Autodesk Fusion 360 part; units mm, degrees
(part 9 of 10)
equation "d1708 = PegSize + 2 * FitClearance"
equation "d1709 = PegSize + 2 * FitClearance"
equation "d1710 = PegHeight + 0.3 mm"
equation "d1712 = FootHeight"
equation "d1714 = ( BaseX + LeftRun + FaucetGap + RightRun - RightSideDepth ) + ( ( RightSideDepth ) - ( ( ( ( RightSideDepth ) - FrontFootInset ) - PegSize / 2 - FitClearance ) + ( PegSize + 2 * FitClearance ) ) )"
equation "d1715 = ( BaseY + Depth + ModuleGap ) + ( ( 11 mm ) - PegSize / 2 - FitClearance )"
equation "d1716 = PegSize + 2 * FitClearance"
equation "d1717 = PegSize + 2 * FitClearance"
equation "d1718 = PegHeight + 0.3 mm"
equation "d1720 = FootHeight"
equation "d1722 = ( BaseX + LeftRun + FaucetGap + RightRun - RightSideDepth ) + ( ( RightSideDepth ) - ( ( ( 11 mm ) - PegSize / 2 - FitClearance ) + ( PegSize + 2 * FitClearance ) ) )"
equation "d1723 = ( BaseY + Depth + ModuleGap ) + ( ( ( RightReach ) - 11 mm ) - PegSize / 2 - FitClearance )"
equation "d1724 = PegSize + 2 * FitClearance"
equation "d1725 = PegSize + 2 * FitClearance"
equation "d1726 = PegHeight + 0.3 mm"
equation "d1728 = FootHeight"
equation "d1730 = ( BaseX + LeftRun + FaucetGap + RightRun - RightSideDepth ) + ( ( RightSideDepth ) - ( ( ( ( RightSideDepth ) - FrontFootInset ) - PegSize / 2 - FitClearance ) + ( PegSize + 2 * FitClearance ) ) )"
equation "d1731 = ( BaseY + Depth + ModuleGap ) + ( ( ( RightReach ) - 11 mm ) - PegSize / 2 - FitClearance )"
equation "d1732 = PegSize + 2 * FitClearance"
equation "d1733 = PegSize + 2 * FitClearance"
equation "d1734 = PegHeight + 0.3 mm"
equation "d1736 = ( FootHeight ) + PanHeight - DeckThick"
equation "d1738 = ( BaseX + LeftRun + FaucetGap + RightRun - RightSideDepth ) + ( ( RightSideDepth ) - ( ( Wall + DeckClearance ) + ( ( RightSideDepth ) - 2 * ( Wall + DeckClearance ) ) ) )"
equation "d1739 = ( BaseY + Depth + ModuleGap ) + ( Wall + DeckClearance )"
equation "d1740 = ( RightSideDepth ) - 2 * ( Wall + DeckClearance )"
equation "d1741 = ( RightReach ) - 2 * ( Wall + DeckClearance )"
equation "d1742 = DeckThick"
equation "d1744 = ( FootHeight ) + PanHeight - DeckThick"
equation "d1746 = ( BaseX + LeftRun + FaucetGap + RightRun - RightSideDepth ) + ( ( RightSideDepth ) - ( ( Wall + DeckClearance + RimBorder ) + ( ( RightSideDepth ) - 2 * ( Wall + DeckClearance + RimBorder ) ) ) )"
equation "d1747 = ( BaseY + Depth + ModuleGap ) + ( ( ( ( RightReach ) - ( 14 * SlotPitch + SlotWidth ) ) / 2 ) + ( 0 * SlotPitch ) )"
equation "d1748 = ( RightSideDepth ) - 2 * ( Wall + DeckClearance + RimBorder )"
equation "d1749 = SlotWidth"
equation "d1750 = DeckThick"
equation "d1752 = ( FootHeight ) + PanHeight - DeckThick"
equation "d1754 = ( BaseX + LeftRun + FaucetGap + RightRun - RightSideDepth ) + ( ( RightSideDepth ) - ( ( Wall + DeckClearance + RimBorder ) + ( ( RightSideDepth ) - 2 * ( Wall + DeckClearance + RimBorder ) ) ) )"
equation "d1755 = ( BaseY + Depth + ModuleGap ) + ( ( ( ( RightReach ) - ( 14 * SlotPitch + SlotWidth ) ) / 2 ) + ( 1 * SlotPitch ) )"
equation "d1756 = ( RightSideDepth ) - 2 * ( Wall + DeckClearance + RimBorder )"
equation "d1757 = SlotWidth"
equation "d1758 = DeckThick"
equation "d1760 = ( FootHeight ) + PanHeight - DeckThick"
equation "d1762 = ( BaseX + LeftRun + FaucetGap + RightRun - RightSideDepth ) + ( ( RightSideDepth ) - ( ( Wall + DeckClearance + RimBorder ) + ( ( RightSideDepth ) - 2 * ( Wall + DeckClearance + RimBorder ) ) ) )"
equation "d1763 = ( BaseY + Depth + ModuleGap ) + ( ( ( ( RightReach ) - ( 14 * SlotPitch + SlotWidth ) ) / 2 ) + ( 2 * SlotPitch ) )"
equation "d1764 = ( RightSideDepth ) - 2 * ( Wall + DeckClearance + RimBorder )"
equation "d1765 = SlotWidth"
equation "d1766 = DeckThick"
equation "d1768 = ( FootHeight ) + PanHeight - DeckThick"
equation "d1770 = ( BaseX + LeftRun + FaucetGap + RightRun - RightSideDepth ) + ( ( RightSideDepth ) - ( ( Wall + DeckClearance + RimBorder ) + ( ( RightSideDepth ) - 2 * ( Wall + DeckClearance + RimBorder ) ) ) )"
equation "d1771 = ( BaseY + Depth + ModuleGap ) + ( ( ( ( RightReach ) - ( 14 * SlotPitch + SlotWidth ) ) / 2 ) + ( 3 * SlotPitch ) )"
equation "d1772 = ( RightSideDepth ) - 2 * ( Wall + DeckClearance + RimBorder )"
equation "d1773 = SlotWidth"
equation "d1774 = DeckThick"
equation "d1776 = ( FootHeight ) + PanHeight - DeckThick"
equation "d1778 = ( BaseX + LeftRun + FaucetGap + RightRun - RightSideDepth ) + ( ( RightSideDepth ) - ( ( Wall + DeckClearance + RimBorder ) + ( ( RightSideDepth ) - 2 * ( Wall + DeckClearance + RimBorder ) ) ) )"
equation "d1779 = ( BaseY + Depth + ModuleGap ) + ( ( ( ( RightReach ) - ( 14 * SlotPitch + SlotWidth ) ) / 2 ) + ( 4 * SlotPitch ) )"
equation "d1780 = ( RightSideDepth ) - 2 * ( Wall + DeckClearance + RimBorder )"
equation "d1781 = SlotWidth"
equation "d1782 = DeckThick"
equation "d1784 = ( FootHeight ) + PanHeight - DeckThick"
equation "d1786 = ( BaseX + LeftRun + FaucetGap + RightRun - RightSideDepth ) + ( ( RightSideDepth ) - ( ( Wall + DeckClearance + RimBorder ) + ( ( RightSideDepth ) - 2 * ( Wall + DeckClearance + RimBorder ) ) ) )"
equation "d1787 = ( BaseY + Depth + ModuleGap ) + ( ( ( ( RightReach ) - ( 14 * SlotPitch + SlotWidth ) ) / 2 ) + ( 5 * SlotPitch ) )"
equation "d1788 = ( RightSideDepth ) - 2 * ( Wall + DeckClearance + RimBorder )"
equation "d1789 = SlotWidth"
equation "d1790 = DeckThick"
equation "d1792 = ( FootHeight ) + PanHeight - DeckThick"
equation "d1794 = ( BaseX + LeftRun + FaucetGap + RightRun - RightSideDepth ) + ( ( RightSideDepth ) - ( ( Wall + DeckClearance + RimBorder ) + ( ( RightSideDepth ) - 2 * ( Wall + DeckClearance + RimBorder ) ) ) )"
equation "d1795 = ( BaseY + Depth + ModuleGap ) + ( ( ( ( RightReach ) - ( 14 * SlotPitch + SlotWidth ) ) / 2 ) + ( 6 * SlotPitch ) )"
equation "d1796 = ( RightSideDepth ) - 2 * ( Wall + DeckClearance + RimBorder )"
equation "d1797 = SlotWidth"
equation "d1798 = DeckThick"
equation "d1800 = ( FootHeight ) + PanHeight - DeckThick"
equation "d1802 = ( BaseX + LeftRun + FaucetGap + RightRun - RightSideDepth ) + ( ( RightSideDepth ) - ( ( Wall + DeckClearance + RimBorder ) + ( ( RightSideDepth ) - 2 * ( Wall + DeckClearance + RimBorder ) ) ) )"
equation "d1803 = ( BaseY + Depth + ModuleGap ) + ( ( ( ( RightReach ) - ( 14 * SlotPitch + SlotWidth ) ) / 2 ) + ( 7 * SlotPitch ) )"
equation "d1804 = ( RightSideDepth ) - 2 * ( Wall + DeckClearance + RimBorder )"
equation "d1805 = SlotWidth"
equation "d1806 = DeckThick"
equation "d1808 = ( FootHeight ) + PanHeight - DeckThick"
equation "d1810 = ( BaseX + LeftRun + FaucetGap + RightRun - RightSideDepth ) + ( ( RightSideDepth ) - ( ( Wall + DeckClearance + RimBorder ) + ( ( RightSideDepth ) - 2 * ( Wall + DeckClearance + RimBorder ) ) ) )"
equation "d1811 = ( BaseY + Depth + ModuleGap ) + ( ( ( ( RightReach ) - ( 14 * SlotPitch + SlotWidth ) ) / 2 ) + ( 8 * SlotPitch ) )"
equation "d1812 = ( RightSideDepth ) - 2 * ( Wall + DeckClearance + RimBorder )"
equation "d1813 = SlotWidth"
equation "d1814 = DeckThick"
equation "d1816 = ( FootHeight ) + PanHeight - DeckThick"
equation "d1818 = ( BaseX + LeftRun + FaucetGap + RightRun - RightSideDepth ) + ( ( RightSideDepth ) - ( ( Wall + DeckClearance + RimBorder ) + ( ( RightSideDepth ) - 2 * ( Wall + DeckClearance + RimBorder ) ) ) )"
equation "d1819 = ( BaseY + Depth + ModuleGap ) + ( ( ( ( RightReach ) - ( 14 * SlotPitch + SlotWidth ) ) / 2 ) + ( 9 * SlotPitch ) )"
equation "d1820 = ( RightSideDepth ) - 2 * ( Wall + DeckClearance + RimBorder )"
equation "d1821 = SlotWidth"
equation "d1822 = DeckThick"
equation "d1824 = ( FootHeight ) + PanHeight - DeckThick"
equation "d1826 = ( BaseX + LeftRun + FaucetGap + RightRun - RightSideDepth ) + ( ( RightSideDepth ) - ( ( Wall + DeckClearance + RimBorder ) + ( ( RightSideDepth ) - 2 * ( Wall + DeckClearance + RimBorder ) ) ) )"
equation "d1827 = ( BaseY + Depth + ModuleGap ) + ( ( ( ( RightReach ) - ( 14 * SlotPitch + SlotWidth ) ) / 2 ) + ( 10 * SlotPitch ) )"
equation "d1828 = ( RightSideDepth ) - 2 * ( Wall + DeckClearance + RimBorder )"
equation "d1829 = SlotWidth"
equation "d1830 = DeckThick"
equation "d1832 = ( FootHeight ) + PanHeight - DeckThick"
equation "d1834 = ( BaseX + LeftRun + FaucetGap + RightRun - RightSideDepth ) + ( ( RightSideDepth ) - ( ( Wall + DeckClearance + RimBorder ) + ( ( RightSideDepth ) - 2 * ( Wall + DeckClearance + RimBorder ) ) ) )"
equation "d1835 = ( BaseY + Depth + ModuleGap ) + ( ( ( ( RightReach ) - ( 14 * SlotPitch + SlotWidth ) ) / 2 ) + ( 11 * SlotPitch ) )"
equation "d1836 = ( RightSideDepth ) - 2 * ( Wall + DeckClearance + RimBorder )"
equation "d1837 = SlotWidth"
equation "d1838 = DeckThick"
equation "d1840 = ( FootHeight ) + PanHeight - DeckThick"
equation "d1842 = ( BaseX + LeftRun + FaucetGap + RightRun - RightSideDepth ) + ( ( RightSideDepth ) - ( ( Wall + DeckClearance + RimBorder ) + ( ( RightSideDepth ) - 2 * ( Wall + DeckClearance + RimBorder ) ) ) )"
equation "d1843 = ( BaseY + Depth + ModuleGap ) + ( ( ( ( RightReach ) - ( 14 * SlotPitch + SlotWidth ) ) / 2 ) + ( 12 * SlotPitch ) )"
equation "d1844 = ( RightSideDepth ) - 2 * ( Wall + DeckClearance + RimBorder )"
equation "d1845 = SlotWidth"
equation "d1846 = DeckThick"
equation "d1848 = ( FootHeight ) + PanHeight - DeckThick"
equation "d1850 = ( BaseX + LeftRun + FaucetGap + RightRun - RightSideDepth ) + ( ( RightSideDepth ) - ( ( Wall + DeckClearance + RimBorder ) + ( ( RightSideDepth ) - 2 * ( Wall + DeckClearance + RimBorder ) ) ) )"
equation "d1851 = ( BaseY + Depth + ModuleGap ) + ( ( ( ( RightReach ) - ( 14 * SlotPitch + SlotWidth ) ) / 2 ) + ( 13 * SlotPitch ) )"
equation "d1852 = ( RightSideDepth ) - 2 * ( Wall + DeckClearance + RimBorder )"
equation "d1853 = SlotWidth"
equation "d1854 = DeckThick"
equation "d1856 = ( FootHeight ) + PanHeight - DeckThick"
equation "d1858 = ( BaseX + LeftRun + FaucetGap + RightRun - RightSideDepth ) + ( ( RightSideDepth ) - ( ( Wall + DeckClearance + RimBorder ) + ( ( RightSideDepth ) - 2 * ( Wall + DeckClearance + RimBorder ) ) ) )"
equation "d1859 = ( BaseY + Depth + ModuleGap ) + ( ( ( ( RightReach ) - ( 14 * SlotPitch + SlotWidth ) ) / 2 ) + ( 14 * SlotPitch ) )"
equation "d1860 = ( RightSideDepth ) - 2 * ( Wall + DeckClearance + RimBorder )"
equation "d1861 = SlotWidth"
equation "d1862 = DeckThick"
equation "d1864 = ( FootHeight ) + PanHeight - DeckThick"
equation "d1866 = ( BaseX + LeftRun + FaucetGap + RightRun - RightSideDepth ) + ( ( RightSideDepth ) - ( ( ( RightSideDepth ) - Wall - DeckClearance - 4 mm ) + ( 5 mm ) ) )"
equation "d1867 = ( BaseY + Depth + ModuleGap ) + ( ( RightReach ) / 2 - 8 mm )"
equation "d1870 = DeckThick"
equation "d1874 = ( BaseX + LeftRun + FaucetGap + RightRun - RightSideDepth ) + ( ( RightSideDepth ) - ( ( ( 11 mm ) - FootSize / 2 ) + ( FootSize ) ) )"
equation "d1875 = ( BaseY + Depth + ModuleGap ) + ( ( 11 mm ) - FootSize / 2 )"
equation "d1876 = FootSize"
equation "d1877 = FootSize"
equation "d1878 = FootHeight"
equation "d1880 = FootHeight"
equation "d1882 = ( BaseX + LeftRun + FaucetGap + RightRun - RightSideDepth ) + ( ( RightSideDepth ) - ( ( ( 11 mm ) - PegSize / 2 ) + ( PegSize ) ) )"
equation "d1883 = ( BaseY + Depth + ModuleGap ) + ( ( 11 mm ) - PegSize / 2 )"
equation "d1884 = PegSize"
equation "d1885 = PegSize"
equation "d1886 = PegHeight"
equation "d1890 = ( BaseX + LeftRun + FaucetGap + RightRun - RightSideDepth ) + ( ( RightSideDepth ) - ( ( ( ( RightSideDepth ) - FrontFootInset ) - FootSize / 2 ) + ( FootSize ) ) )"
equation "d1891 = ( BaseY + Depth + ModuleGap ) + ( ( 11 mm ) - FootSize / 2 )"
equation "d1892 = FootSize"
equation "d1893 = FootSize"
equation "d1894 = FootHeight"
equation "d1896 = FootHeight"
equation "d1898 = ( BaseX + LeftRun + FaucetGap + RightRun - RightSideDepth ) + ( ( RightSideDepth ) - ( ( ( ( RightSideDepth ) - FrontFootInset ) - PegSize / 2 ) + ( PegSize ) ) )"
equation "d1899 = ( BaseY + Depth + ModuleGap ) + ( ( 11 mm ) - PegSize / 2 )"
equation "d1900 = PegSize"
equation "d1901 = PegSize"
equation "d1902 = PegHeight"
equation "d1906 = ( BaseX + LeftRun + FaucetGap + RightRun - RightSideDepth ) + ( ( RightSideDepth ) - ( ( ( 11 mm ) - FootSize / 2 ) + ( FootSize ) ) )"
equation "d1907 = ( BaseY + Depth + ModuleGap ) + ( ( ( RightReach ) - 11 mm ) - FootSize / 2 )"
equation "d1908 = FootSize"
equation "d1909 = FootSize"
equation "d1910 = FootHeight"
equation "d1912 = FootHeight"
equation "d1914 = ( BaseX + LeftRun + FaucetGap + RightRun - RightSideDepth ) + ( ( RightSideDepth ) - ( ( ( 11 mm ) - PegSize / 2 ) + ( PegSize ) ) )"
equation "d1915 = ( BaseY + Depth + ModuleGap ) + ( ( ( RightReach ) - 11 mm ) - PegSize / 2 )"
equation "d1916 = PegSize"
equation "d1917 = PegSize"
equation "d1918 = PegHeight"
equation "d1922 = ( BaseX + LeftRun + FaucetGap + RightRun - RightSideDepth ) + ( ( RightSideDepth ) - ( ( ( ( RightSideDepth ) - FrontFootInset ) - FootSize / 2 ) + ( FootSize ) ) )"
equation "d1923 = ( BaseY + Depth + ModuleGap ) + ( ( ( RightReach ) - 11 mm ) - FootSize / 2 )"
equation "d1924 = FootSize"
equation "d1925 = FootSize"
equation "d1926 = FootHeight"
equation "d1928 = FootHeight"
equation "d1930 = ( BaseX + LeftRun + FaucetGap + RightRun - RightSideDepth ) + ( ( RightSideDepth ) - ( ( ( ( RightSideDepth ) - FrontFootInset ) - PegSize / 2 ) + ( PegSize ) ) )"
equation "d1931 = ( BaseY + Depth + ModuleGap ) + ( ( ( RightReach ) - 11 mm ) - PegSize / 2 )"
equation "d1932 = PegSize"
equation "d1933 = PegSize"
equation "d1934 = PegHeight"
equation "d1936 = UpperDeckHeight - PanHeight"
equation "d1938 = ( BaseX ) + ( 0 mm )"
equation "d1939 = ( BaseY ) + ( 0 mm )"
equation "d1940 = TowerWidth"
equation "d1941 = Depth"
equation "d1942 = PanHeight"
equation "d1946 = ( BaseX ) + ( Wall )"
equation "d1948 = -( -( ( UpperDeckHeight - PanHeight ) + FloorMin + DrainExtension * tan(DrainSlope) + ( ( Depth ) - ( Wall ) ) * tan(DrainSlope) ) )"
equation "d1949 = ( ( BaseY ) + ( Wall ) )"
equation "d1950 = -( -( ( UpperDeckHeight - PanHeight ) + FloorMin + DrainExtension * tan(DrainSlope) + ( ( Depth ) - ( ( Depth ) - Wall ) ) * tan(DrainSlope) ) )"
equation "d1951 = ( ( BaseY ) + ( ( Depth ) - Wall ) )"
equation "d1952 = -( -( ( UpperDeckHeight - PanHeight ) + PanHeight + 1 mm ) )"
equation "d1953 = ( TowerWidth ) - 2 * Wall"
equation "d1955 = ( BaseX ) + ( ( TowerWidth - 35 mm ) - DrainWidth / 2 - Wall )"
equation "d1957 = -( -( UpperDeckHeight - PanHeight ) )"
equation "d1958 = ( ( BaseY ) + ( ( Depth ) - Wall ) )"
equation "d1959 = ( ( BaseY ) + ( ( Depth ) + DrainExtension ) )"
equation "d1960 = -( -( ( UpperDeckHeight - PanHeight ) + FloorMin + DrainExtension * tan(DrainSlope) + ( ( Depth ) - ( ( Depth ) + DrainExtension ) ) * tan(DrainSlope) ) )"
equation "d1961 = -( -( ( UpperDeckHeight - PanHeight ) + FloorMin + DrainExtension * tan(DrainSlope) + ( ( Depth ) - ( ( Depth ) - Wall ) ) * tan(DrainSlope) ) )"
equation "d1962 = DrainWidth + 2 * Wall"
equation "d1964 = ( BaseX ) + ( ( TowerWidth - 35 mm ) - DrainWidth / 2 - Wall )"
equation "d1966 = -( -( UpperDeckHeight - PanHeight ) )"
equation "d1967 = ( ( BaseY ) + ( ( Depth ) - Wall ) )"
equation "d1968 = ( ( BaseY ) + ( ( Depth ) + DrainExtension ) )"
equation "d1969 = -( -( ( ( UpperDeckHeight - PanHeight ) + FloorMin + DrainExtension * tan(DrainSlope) + ( ( Depth ) - ( ( Depth ) + DrainExtension ) ) * tan(DrainSlope) ) + ( 6 mm ) ) )"
equation "d1970 = -( -( ( ( UpperDeckHeight - PanHeight ) + FloorMin + DrainExtension * tan(DrainSlope) + ( ( Depth ) - ( ( Depth ) - Wall ) ) * tan(DrainSlope) ) + ( 6 mm ) ) )"
equation "d1971 = Wall"
equation "d1973 = ( BaseX ) + ( ( TowerWidth - 35 mm ) + DrainWidth / 2 )"
equation "d1975 = -( -( UpperDeckHeight - PanHeight ) )"
equation "d1976 = ( ( BaseY ) + ( ( Depth ) - Wall ) )"
equation "d1977 = ( ( BaseY ) + ( ( Depth ) + DrainExtension ) )"
equation "d1978 = -( -( ( ( UpperDeckHeight - PanHeight ) + FloorMin + DrainExtension * tan(DrainSlope) + ( ( Depth ) - ( ( Depth ) + DrainExtension ) ) * tan(DrainSlope) ) + ( 6 mm ) ) )"
equation "d1979 = -( -( ( ( UpperDeckHeight - PanHeight ) + FloorMin + DrainExtension * tan(DrainSlope) + ( ( Depth ) - ( ( Depth ) - Wall ) ) * tan(DrainSlope) ) + ( 6 mm ) ) )"
equation "d1980 = Wall"
equation "d1982 = ( BaseX ) + ( ( TowerWidth - 35 mm ) - DrainWidth / 2 )"
equation "d1984 = -( -( ( UpperDeckHeight - PanHeight ) + FloorMin + DrainExtension * tan(DrainSlope) + ( ( Depth ) - ( ( Depth ) - Wall ) ) * tan(DrainSlope) ) )"
equation "d1985 = ( ( BaseY ) + ( ( Depth ) - Wall ) )"
equation "d1986 = -( -( ( UpperDeckHeight - PanHeight ) + FloorMin + DrainExtension * tan(DrainSlope) + ( ( Depth ) - ( ( Depth ) + DrainExtension ) ) * tan(DrainSlope) ) )"
equation "d1987 = ( ( BaseY ) + ( ( Depth ) + DrainExtension ) )"
equation "d1988 = -( -( ( UpperDeckHeight - PanHeight ) + PanHeight + 1 mm ) )"
equation "d1989 = DrainWidth"
equation "d1991 = UpperDeckHeight - PanHeight"
equation "d1993 = ( BaseX ) + ( Wall )"
equation "d1994 = ( BaseY ) + ( Wall )"
equation "d1997 = PanHeight - DeckThick"
equation "d1999 = UpperDeckHeight - PanHeight"
equation "d2001 = ( BaseX ) + ( Wall )"
equation "d2002 = ( BaseY ) + ( ( Depth ) - Wall - 12 mm )"
equation "d2005 = PanHeight - DeckThick"
equation "d2007 = UpperDeckHeight - PanHeight"
equation "d2009 = ( BaseX ) + ( ( TowerWidth ) - Wall - 12 mm )"
equation "d2010 = ( BaseY ) + ( Wall )"
equation "d2013 = PanHeight - DeckThick"
equation "d2015 = UpperDeckHeight - PanHeight"
equation "d2017 = ( BaseX ) + ( ( TowerWidth ) - Wall - 12 mm )"
equation "d2018 = ( BaseY ) + ( ( Depth ) - Wall - 12 mm )"
equation "d2021 = PanHeight - DeckThick"
equation "d2023 = ( BaseX ) + ( ( TowerWidth - 35 mm ) - DrainWidth / 2 - Wall )"
equation "d2025 = -( -( ( UpperDeckHeight - PanHeight ) - ( 0.2 mm ) ) )"
equation "d2026 = ( ( BaseY ) + ( ( Depth ) + DrainExtension - 2 mm ) )"
equation "d2027 = ( ( BaseY ) + ( ( ( Depth ) + DrainExtension - 2 mm ) + ( 1 mm ) ) )"
equation "d2028 = -( -( ( UpperDeckHeight - PanHeight ) + ( 0.6 mm ) ) )"
equation "d2029 = DrainWidth + 2 * Wall"
equation "d2031 = ( UpperDeckHeight - PanHeight ) + PanHeight - DeckThick"
equation "d2033 = ( BaseX ) + ( Wall + DeckClearance )"
equation "d2034 = ( BaseY ) + ( Wall + DeckClearance )"
equation "d2035 = ( TowerWidth ) - 2 * ( Wall + DeckClearance )"
equation "d2036 = ( Depth ) - 2 * ( Wall + DeckClearance )"
equation "d2037 = DeckThick"
equation "d2039 = ( UpperDeckHeight - PanHeight ) + PanHeight - DeckThick"
equation "d2041 = ( BaseX ) + ( ( ( ( TowerWidth ) - ( 14 * SlotPitch + SlotWidth ) ) / 2 ) + ( 0 * SlotPitch ) )"
equation "d2042 = ( BaseY ) + ( Wall + DeckClearance + RimBorder )"
equation "d2043 = SlotWidth"
equation "d2044 = ( Depth ) - 2 * ( Wall + DeckClearance + RimBorder )"
equation "d2045 = DeckThick"
equation "d2047 = ( UpperDeckHeight - PanHeight ) + PanHeight - DeckThick"
equation "d2049 = ( BaseX ) + ( ( ( ( TowerWidth ) - ( 14 * SlotPitch + SlotWidth ) ) / 2 ) + ( 1 * SlotPitch ) )"
equation "d2050 = ( BaseY ) + ( Wall + DeckClearance + RimBorder )"
equation "d2051 = SlotWidth"
equation "d2052 = ( Depth ) - 2 * ( Wall + DeckClearance + RimBorder )"
equation "d2053 = DeckThick"
equation "d2055 = ( UpperDeckHeight - PanHeight ) + PanHeight - DeckThick"
equation "d2057 = ( BaseX ) + ( ( ( ( TowerWidth ) - ( 14 * SlotPitch + SlotWidth ) ) / 2 ) + ( 2 * SlotPitch ) )"
equation "d2058 = ( BaseY ) + ( Wall + DeckClearance + RimBorder )"
equation "d2059 = SlotWidth"
equation "d2060 = ( Depth ) - 2 * ( Wall + DeckClearance + RimBorder )"
equation "d2061 = DeckThick"
equation "d2063 = ( UpperDeckHeight - PanHeight ) + PanHeight - DeckThick"
equation "d2065 = ( BaseX ) + ( ( ( ( TowerWidth ) - ( 14 * SlotPitch + SlotWidth ) ) / 2 ) + ( 3 * SlotPitch ) )"
equation "d2066 = ( BaseY ) + ( Wall + DeckClearance + RimBorder )"
equation "d2067 = SlotWidth"
equation "d2068 = ( Depth ) - 2 * ( Wall + DeckClearance + RimBorder )"
equation "d2069 = DeckThick"
equation "d2071 = ( UpperDeckHeight - PanHeight ) + PanHeight - DeckThick"
equation "d2073 = ( BaseX ) + ( ( ( ( TowerWidth ) - ( 14 * SlotPitch + SlotWidth ) ) / 2 ) + ( 4 * SlotPitch ) )"
equation "d2074 = ( BaseY ) + ( Wall + DeckClearance + RimBorder )"
equation "d2075 = SlotWidth"
equation "d2076 = ( Depth ) - 2 * ( Wall + DeckClearance + RimBorder )"
equation "d2077 = DeckThick"
equation "d2079 = ( UpperDeckHeight - PanHeight ) + PanHeight - DeckThick"
equation "d2081 = ( BaseX ) + ( ( ( ( TowerWidth ) - ( 14 * SlotPitch + SlotWidth ) ) / 2 ) + ( 5 * SlotPitch ) )"
equation "d2082 = ( BaseY ) + ( Wall + DeckClearance + RimBorder )"
equation "d2083 = SlotWidth"
equation "d2084 = ( Depth ) - 2 * ( Wall + DeckClearance + RimBorder )"
equation "d2085 = DeckThick"
equation "d2087 = ( UpperDeckHeight - PanHeight ) + PanHeight - DeckThick"
equation "d2089 = ( BaseX ) + ( ( ( ( TowerWidth ) - ( 14 * SlotPitch + SlotWidth ) ) / 2 ) + ( 6 * SlotPitch ) )"
equation "d2090 = ( BaseY ) + ( Wall + DeckClearance + RimBorder )"
equation "d2091 = SlotWidth"
equation "d2092 = ( Depth ) - 2 * ( Wall + DeckClearance + RimBorder )"
equation "d2093 = DeckThick"
equation "d2095 = ( UpperDeckHeight - PanHeight ) + PanHeight - DeckThick"
equation "d2097 = ( BaseX ) + ( ( ( ( TowerWidth ) - ( 14 * SlotPitch + SlotWidth ) ) / 2 ) + ( 7 * SlotPitch ) )"
equation "d2098 = ( BaseY ) + ( Wall + DeckClearance + RimBorder )"
equation "d2099 = SlotWidth"
equation "d2100 = ( Depth ) - 2 * ( Wall + DeckClearance + RimBorder )"
equation "d2101 = DeckThick"
equation "d2103 = ( UpperDeckHeight - PanHeight ) + PanHeight - DeckThick"
equation "d2105 = ( BaseX ) + ( ( ( ( TowerWidth ) - ( 14 * SlotPitch + SlotWidth ) ) / 2 ) + ( 8 * SlotPitch ) )"
equation "d2106 = ( BaseY ) + ( Wall + DeckClearance + RimBorder )"
equation "d2107 = SlotWidth"
equation "d2108 = ( Depth ) - 2 * ( Wall + DeckClearance + RimBorder )"
equation "d2109 = DeckThick"
equation "d2111 = ( UpperDeckHeight - PanHeight ) + PanHeight - DeckThick"
equation "d2113 = ( BaseX ) + ( ( ( ( TowerWidth ) - ( 14 * SlotPitch + SlotWidth ) ) / 2 ) + ( 9 * SlotPitch ) )"
equation "d2114 = ( BaseY ) + ( Wall + DeckClearance + RimBorder )"
equation "d2115 = SlotWidth"
equation "d2116 = ( Depth ) - 2 * ( Wall + DeckClearance + RimBorder )"
equation "d2117 = DeckThick"
equation "d2119 = ( UpperDeckHeight - PanHeight ) + PanHeight - DeckThick"
equation "d2121 = ( BaseX ) + ( ( ( ( TowerWidth ) - ( 14 * SlotPitch + SlotWidth ) ) / 2 ) + ( 10 * SlotPitch ) )"
equation "d2122 = ( BaseY ) + ( Wall + DeckClearance + RimBorder )"
equation "d2123 = SlotWidth"
equation "d2124 = ( Depth ) - 2 * ( Wall + DeckClearance + RimBorder )"
equation "d2125 = DeckThick"
equation "d2127 = ( UpperDeckHeight - PanHeight ) + PanHeight - DeckThick"
equation "d2129 = ( BaseX ) + ( ( ( ( TowerWidth ) - ( 14 * SlotPitch + SlotWidth ) ) / 2 ) + ( 11 * SlotPitch ) )"
equation "d2130 = ( BaseY ) + ( Wall + DeckClearance + RimBorder )"
equation "d2131 = SlotWidth"
equation "d2132 = ( Depth ) - 2 * ( Wall + DeckClearance + RimBorder )"
equation "d2133 = DeckThick"
equation "d2135 = ( UpperDeckHeight - PanHeight ) + PanHeight - DeckThick"
equation "d2137 = ( BaseX ) + ( ( ( ( TowerWidth ) - ( 14 * SlotPitch + SlotWidth ) ) / 2 ) + ( 12 * SlotPitch ) )"
equation "d2138 = ( BaseY ) + ( Wall + DeckClearance + RimBorder )"
equation "d2139 = SlotWidth"
equation "d2140 = ( Depth ) - 2 * ( Wall + DeckClearance + RimBorder )"
equation "d2141 = DeckThick"
equation "d2143 = ( UpperDeckHeight - PanHeight ) + PanHeight - DeckThick"
equation "d2145 = ( BaseX ) + ( ( ( ( TowerWidth ) - ( 14 * SlotPitch + SlotWidth ) ) / 2 ) + ( 13 * SlotPitch ) )"
equation "d2146 = ( BaseY ) + ( Wall + DeckClearance + RimBorder )"
equation "d2147 = SlotWidth"
equation "d2148 = ( Depth ) - 2 * ( Wall + DeckClearance + RimBorder )"
equation "d2149 = DeckThick"
equation "d2151 = ( UpperDeckHeight - PanHeight ) + PanHeight - DeckThick"
equation "d2153 = ( BaseX ) + ( ( ( ( TowerWidth ) - ( 14 * SlotPitch + SlotWidth ) ) / 2 ) + ( 14 * SlotPitch ) )"
equation "d2154 = ( BaseY ) + ( Wall + DeckClearance + RimBorder )"
equation "d2155 = SlotWidth"
equation "d2156 = ( Depth ) - 2 * ( Wall + DeckClearance + RimBorder )"
equation "d2157 = DeckThick"
equation "d2159 = ( UpperDeckHeight - PanHeight ) + PanHeight - DeckThick"
equation "d2161 = ( BaseX ) + ( ( TowerWidth ) / 2 - 8 mm )"
equation "d2162 = ( BaseY ) + ( ( Depth ) - Wall - DeckClearance - 4 mm )"
equation "d2165 = DeckThick"
equation "d2169 = BaseX"
equation "d2170 = BaseY"
equation "d2171 = TowerFrame"
equation "d2172 = Depth"
equation "d2173 = UpperDeckHeight - PanHeight"
equation "d2175 = BaseX"
equation "d2177 = -( -( 8 mm ) )"
equation "d2178 = ( BaseY + 12 mm )"
equation "d2179 = ( BaseY + Depth - 12 mm )"
equation "d2180 = -( -( UpperDeckHeight - PanHeight - 8 mm ) )"
equation "d2181 = TowerFrame"
equation "d2183 = UpperDeckHeight - PanHeight"
equation "d2185 = ( BaseX ) + ( ( TowerFrame - 5 mm ) / 2 )"
equation "d2186 = ( BaseY + 8 mm ) - ( 2.5 mm )"
equation "d2189 = PegHeight"
equation "d2191 = UpperDeckHeight - PanHeight"
equation "d2193 = ( BaseX ) + ( ( TowerFrame - 5 mm ) / 2 )"
equation "d2194 = ( BaseY + Depth - 8 mm ) - ( 2.5 mm )"
equation "d2197 = PegHeight"
equation "d2201 = BaseX + TowerWidth - TowerFrame"
equation "d2202 = BaseY"
equation "d2203 = TowerFrame"
equation "d2204 = Depth"
equation "d2205 = UpperDeckHeight - PanHeight"
equation "d2207 = BaseX + TowerWidth - TowerFrame"
equation "d2209 = -( -( 8 mm ) )"
equation "d2210 = ( BaseY + 12 mm )"
equation "d2211 = ( BaseY + Depth - 12 mm )"
equation "d2212 = -( -( UpperDeckHeight - PanHeight - 8 mm ) )"
equation "d2213 = TowerFrame"
equation "d2215 = UpperDeckHeight - PanHeight"
equation "d2217 = ( BaseX + TowerWidth - TowerFrame ) + ( ( TowerFrame - 5 mm ) / 2 )"
equation "d2218 = ( BaseY + 8 mm ) - ( 2.5 mm )"
equation "d2221 = PegHeight"
equation "d2223 = UpperDeckHeight - PanHeight"
equation "d2225 = ( BaseX + TowerWidth - TowerFrame ) + ( ( TowerFrame - 5 mm ) / 2 )"
equation "d2226 = ( BaseY + Depth - 8 mm ) - ( 2.5 mm )"
equation "d2229 = PegHeight"
equation "d2231 = UpperDeckHeight - PanHeight"
equation "d2233 = ( BaseX + ( TowerFrame - 5 mm ) / 2 ) - ( FitClearance )"
equation "d2234 = ( BaseY + 8 mm ) - ( 2.5 mm + FitClearance )"
equation "d2235 = 5 mm + 2 * FitClearance"
equation "d2236 = 5 mm + 2 * FitClearance"
equation "d2237 = PegHeight + 0.3 mm"
equation "d2239 = UpperDeckHeight - PanHeight"
equation "d2241 = ( BaseX + ( TowerFrame - 5 mm ) / 2 ) - ( FitClearance )"
equation "d2242 = ( BaseY + Depth - 8 mm ) - ( 2.5 mm + FitClearance )"
equation "d2243 = 5 mm + 2 * FitClearance"
equation "d2244 = 5 mm + 2 * FitClearance"
equation "d2245 = PegHeight + 0.3 mm"
equation "d2247 = UpperDeckHeight - PanHeight"
equation "d2249 = ( BaseX + TowerWidth - TowerFrame + ( TowerFrame - 5 mm ) / 2 ) - ( FitClearance )"
equation "d2250 = ( BaseY + 8 mm ) - ( 2.5 mm + FitClearance )"
equation "d2251 = 5 mm + 2 * FitClearance"
equation "d2252 = 5 mm + 2 * FitClearance"
equation "d2253 = PegHeight + 0.3 mm"
equation "d2255 = UpperDeckHeight - PanHeight"
equation "d2257 = ( BaseX + TowerWidth - TowerFrame + ( TowerFrame - 5 mm ) / 2 ) - ( FitClearance )"
equation "d2258 = ( BaseY + Depth - 8 mm ) - ( 2.5 mm + FitClearance )"
equation "d2259 = 5 mm + 2 * FitClearance"
equation "d2260 = 5 mm + 2 * FitClearance"
equation "d2261 = PegHeight + 0.3 mm"
equation "d2265 = BaseX + LeftRun + FaucetGap + RightRun + 20 mm + 0 mm"
equation "d2266 = BaseY"
equation "d2273 = ( BaseX + LeftRun + FaucetGap + RightRun + 20 mm + 0 mm ) + ( ( 24 mm - ( PegSize + 2 * ( FitClearance - 0.05 mm ) ) ) / 2 )"
equation "d2274 = BaseY + ( 24 mm - ( PegSize + 2 * ( FitClearance - 0.05 mm ) ) ) / 2"
equation "d2275 = PegSize + 2 * ( FitClearance - 0.05 mm )"
equation "d2276 = PegSize + 2 * ( FitClearance - 0.05 mm )"
equation "d2277 = PegHeight + 0.3 mm"
equation "d2281 = BaseX + LeftRun + FaucetGap + RightRun + 20 mm + 30 mm"
equation "d2282 = BaseY"
equation "d2289 = ( BaseX + LeftRun + FaucetGap + RightRun + 20 mm + 30 mm ) + ( ( 24 mm - ( PegSize + 2 * ( FitClearance ) ) ) / 2 )"
equation "d2290 = BaseY + ( 24 mm - ( PegSize + 2 * ( FitClearance ) ) ) / 2"
equation "d2291 = PegSize + 2 * ( FitClearance )"
equation "d2292 = PegSize + 2 * ( FitClearance )"
equation "d2293 = PegHeight + 0.3 mm"
equation "d2297 = BaseX + LeftRun + FaucetGap + RightRun + 20 mm + 60 mm"
equation "d2298 = BaseY"
equation "d2305 = ( BaseX + LeftRun + FaucetGap + RightRun + 20 mm + 60 mm ) + ( ( 24 mm - ( PegSize + 2 * ( FitClearance + 0.05 mm ) ) ) / 2 )"
equation "d2306 = BaseY + ( 24 mm - ( PegSize + 2 * ( FitClearance + 0.05 mm ) ) ) / 2"
equation "d2307 = PegSize + 2 * ( FitClearance + 0.05 mm )"
equation "d2308 = PegSize + 2 * ( FitClearance + 0.05 mm )"
equation "d2309 = PegHeight + 0.3 mm"
equation "FrontFootInset = 17 mm" comment "R02 front foot center inset; outer foot edge is 9 mm behind open lip"
equation "d2312 = ( FootHeight ) - 0.2 mm"
equation "d2314 = ( BaseX + TowerFrame + TowerClearance ) + ( -1 mm )"
equation "d2315 = ( BaseY ) + ( Depth )"
equation "d2316 = ( TowerWidth - 2 * ( TowerFrame + TowerClearance ) ) + 2 mm"
equation "d2317 = DrainExtension + 2 mm"
equation "d2318 = PanHeight + 0.4 mm"
equation "d2320 = ( BaseX + TowerFrame + TowerClearance ) + ( Wall )"
equation "d2322 = -( -( ( FootHeight ) + FloorMin + DrainExtension * tan(DrainSlope) + ( ( Depth ) - ( ( Depth ) - Wall - 0.1 mm ) ) * tan(DrainSlope) ) )"
equation "d2323 = ( ( BaseY ) + ( ( Depth ) - Wall - 0.1 mm ) )"
equation "d2324 = -( -( ( FootHeight ) + FloorMin + DrainExtension * tan(DrainSlope) + ( ( Depth ) - ( ( Depth ) + 1 mm ) ) * tan(DrainSlope) ) )"
equation "d2325 = ( ( BaseY ) + ( ( Depth ) + 1 mm ) )"
equation "d2326 = -( -( ( FootHeight ) + PanHeight + 1 mm ) )"
equation "d2327 = ( TowerWidth - 2 * ( TowerFrame + TowerClearance ) ) - 2 * Wall"
equation "d2329 = ( FootHeight ) + PanHeight - DeckThick"
equation "d2331 = ( BaseX + TowerFrame + TowerClearance ) + ( ( Wall ) - DeckClearance )"
equation "d2332 = ( BaseY ) + ( 10 mm - DeckClearance )"
equation "d2333 = 2 mm + 2 * DeckClearance"
equation "d2334 = 5 mm + 2 * DeckClearance"
equation "d2335 = DeckThick"
equation "d2337 = FootHeight"
equation "d2339 = ( BaseX + TowerFrame + TowerClearance ) + ( Wall )"
equation "d2340 = ( BaseY ) + ( 10 mm )"
equation "d2343 = PanHeight"
equation "d2345 = ( FootHeight ) + PanHeight - DeckThick"
equation "d2347 = ( BaseX + TowerFrame + TowerClearance ) + ( ( ( TowerWidth - 2 * ( TowerFrame + TowerClearance ) ) - Wall - 2 mm ) - DeckClearance )"
equation "d2348 = ( BaseY ) + ( 10 mm - DeckClearance )"
equation "d2349 = 2 mm + 2 * DeckClearance"
equation "d2350 = 5 mm + 2 * DeckClearance"
equation "d2351 = DeckThick"
equation "d2353 = FootHeight"
equation "d2355 = ( BaseX + TowerFrame + TowerClearance ) + ( ( TowerWidth - 2 * ( TowerFrame + TowerClearance ) ) - Wall - 2 mm )"
equation "d2356 = ( BaseY ) + ( 10 mm )"
equation "d2359 = PanHeight"
equation "d2361 = ( FootHeight ) - 0.2 mm"
equation "d2363 = ( BaseX + TowerWidth + ModuleGap ) + ( -1 mm )"
equation "d2364 = ( BaseY ) + ( Depth )"
equation "d2365 = ( LeftRun - TowerWidth - ModuleGap ) + 2 mm"
equation "d2366 = DrainExtension + 2 mm"
equation "d2367 = PanHeight + 0.4 mm"
equation "d2369 = ( BaseX + TowerWidth + ModuleGap ) + ( Wall )"
equation "d2371 = -( -( ( FootHeight ) + FloorMin + DrainExtension * tan(DrainSlope) + ( ( Depth ) - ( ( Depth ) - Wall - 0.1 mm ) ) * tan(DrainSlope) ) )"
equation "d2372 = ( ( BaseY ) + ( ( Depth ) - Wall - 0.1 mm ) )"
equation "d2373 = -( -( ( FootHeight ) + FloorMin + DrainExtension * tan(DrainSlope) + ( ( Depth ) - ( ( Depth ) + 1 mm ) ) * tan(DrainSlope) ) )"
equation "d2374 = ( ( BaseY ) + ( ( Depth ) + 1 mm ) )"
equation "d2375 = -( -( ( FootHeight ) + PanHeight + 1 mm ) )"
equation "d2376 = ( LeftRun - TowerWidth - ModuleGap ) - 2 * Wall"
equation "d2378 = ( FootHeight ) + PanHeight - DeckThick"
equation "d2380 = ( BaseX + TowerWidth + ModuleGap ) + ( ( Wall ) - DeckClearance )"
equation "d2381 = ( BaseY ) + ( 10 mm - DeckClearance )"
equation "d2382 = 2 mm + 2 * DeckClearance"
equation "d2383 = 5 mm + 2 * DeckClearance"
equation "d2384 = DeckThick"
equation "d2386 = FootHeight"
equation "d2388 = ( BaseX + TowerWidth + ModuleGap ) + ( Wall )"
equation "d2389 = ( BaseY ) + ( 10 mm )"
equation "d2392 = PanHeight"
equation "d2394 = ( FootHeight ) + PanHeight - DeckThick"
equation "d2396 = ( BaseX + TowerWidth + ModuleGap ) + ( ( ( LeftRun - TowerWidth - ModuleGap ) - Wall - 2 mm ) - DeckClearance )"
equation "d2397 = ( BaseY ) + ( 10 mm - DeckClearance )"
equation "d2398 = 2 mm + 2 * DeckClearance"
equation "d2399 = 5 mm + 2 * DeckClearance"
equation "d2400 = DeckThick"
equation "d2402 = FootHeight"
equation "d2404 = ( BaseX + TowerWidth + ModuleGap ) + ( ( LeftRun - TowerWidth - ModuleGap ) - Wall - 2 mm )"
equation "d2405 = ( BaseY ) + ( 10 mm )"
equation "d2408 = PanHeight"
equation "d2410 = ( FootHeight ) - 0.2 mm"
equation "d2412 = ( BaseX + LeftRun + FaucetGap ) + ( -1 mm )"
equation "d2413 = ( BaseY ) + ( Depth )"
equation "d2414 = ( ( RightRun - ModuleGap ) / 2 ) + 2 mm"
equation "d2415 = DrainExtension + 2 mm"
equation "d2416 = PanHeight + 0.4 mm"
equation "d2418 = ( BaseX + LeftRun + FaucetGap ) + ( Wall )"
equation "d2420 = -( -( ( FootHeight ) + FloorMin + DrainExtension * tan(DrainSlope) + ( ( Depth ) - ( ( Depth ) - Wall - 0.1 mm ) ) * tan(DrainSlope) ) )"
equation "d2421 = ( ( BaseY ) + ( ( Depth ) - Wall - 0.1 mm ) )"
equation "d2422 = -( -( ( FootHeight ) + FloorMin + DrainExtension * tan(DrainSlope) + ( ( Depth ) - ( ( Depth ) + 1 mm ) ) * tan(DrainSlope) ) )"
equation "d2423 = ( ( BaseY ) + ( ( Depth ) + 1 mm ) )"
equation "d2424 = -( -( ( FootHeight ) + PanHeight + 1 mm ) )"
equation "d2425 = ( ( RightRun - ModuleGap ) / 2 ) - 2 * Wall"
equation "d2427 = ( FootHeight ) + PanHeight - DeckThick"
equation "d2429 = ( BaseX + LeftRun + FaucetGap ) + ( ( Wall ) - DeckClearance )"
equation "d2430 = ( BaseY ) + ( 10 mm - DeckClearance )"
equation "d2431 = 2 mm + 2 * DeckClearance"
equation "d2432 = 5 mm + 2 * DeckClearance"
equation "d2433 = DeckThick"
equation "d2435 = FootHeight"
equation "d2437 = ( BaseX + LeftRun + FaucetGap ) + ( Wall )"
equation "d2438 = ( BaseY ) + ( 10 mm )"
equation "d2441 = PanHeight"
equation "d2443 = ( FootHeight ) + PanHeight - DeckThick"
equation "d2445 = ( BaseX + LeftRun + FaucetGap ) + ( ( ( ( RightRun - ModuleGap ) / 2 ) - Wall - 2 mm ) - DeckClearance )"
equation "d2446 = ( BaseY ) + ( 10 mm - DeckClearance )"
equation "d2447 = 2 mm + 2 * DeckClearance"
equation "d2448 = 5 mm + 2 * DeckClearance"
equation "d2449 = DeckThick"
equation "d2451 = FootHeight"
equation "d2453 = ( BaseX + LeftRun + FaucetGap ) + ( ( ( RightRun - ModuleGap ) / 2 ) - Wall - 2 mm )"
equation "d2454 = ( BaseY ) + ( 10 mm )"
equation "d2457 = PanHeight"
equation "d2459 = ( FootHeight ) - 0.2 mm"
equation "d2461 = ( BaseX + LeftRun + FaucetGap + ( RightRun + ModuleGap ) / 2 ) + ( -1 mm )"
equation "d2462 = ( BaseY ) + ( Depth )"
equation "d2463 = ( ( RightRun - ModuleGap ) / 2 ) + 2 mm"
equation "d2464 = DrainExtension + 2 mm"
equation "d2465 = PanHeight + 0.4 mm"
equation "d2467 = ( BaseX + LeftRun + FaucetGap + ( RightRun + ModuleGap ) / 2 ) + ( Wall )"
equation "d2469 = -( -( ( FootHeight ) + FloorMin + DrainExtension * tan(DrainSlope) + ( ( Depth ) - ( ( Depth ) - Wall - 0.1 mm ) ) * tan(DrainSlope) ) )"
equation "d2470 = ( ( BaseY ) + ( ( Depth ) - Wall - 0.1 mm ) )"
equation "d2471 = -( -( ( FootHeight ) + FloorMin + DrainExtension * tan(DrainSlope) + ( ( Depth ) - ( ( Depth ) + 1 mm ) ) * tan(DrainSlope) ) )"
equation "d2472 = ( ( BaseY ) + ( ( Depth ) + 1 mm ) )"
equation "d2473 = -( -( ( FootHeight ) + PanHeight + 1 mm ) )"
equation "d2474 = ( ( RightRun - ModuleGap ) / 2 ) - 2 * Wall"
equation "d2476 = ( FootHeight ) + PanHeight - DeckThick"
equation "d2478 = ( BaseX + LeftRun + FaucetGap + ( RightRun + ModuleGap ) / 2 ) + ( ( Wall ) - DeckClearance )"
equation "d2479 = ( BaseY ) + ( 10 mm - DeckClearance )"
equation "d2480 = 2 mm + 2 * DeckClearance"
equation "d2481 = 5 mm + 2 * DeckClearance"
equation "d2482 = DeckThick"
equation "d2484 = FootHeight"
equation "d2486 = ( BaseX + LeftRun + FaucetGap + ( RightRun + ModuleGap ) / 2 ) + ( Wall )"
equation "d2487 = ( BaseY ) + ( 10 mm )"
equation "d2490 = PanHeight"
equation "d2492 = ( FootHeight ) + PanHeight - DeckThick"
equation "d2494 = ( BaseX + LeftRun + FaucetGap + ( RightRun + ModuleGap ) / 2 ) + ( ( ( ( RightRun - ModuleGap ) / 2 ) - Wall - 2 mm ) - DeckClearance )"
equation "d2495 = ( BaseY ) + ( 10 mm - DeckClearance )"
equation "d2496 = 2 mm + 2 * DeckClearance"
equation "d2497 = 5 mm + 2 * DeckClearance"
equation "d2498 = DeckThick"
equation "d2500 = FootHeight"
equation "d2502 = ( BaseX + LeftRun + FaucetGap + ( RightRun + ModuleGap ) / 2 ) + ( ( ( RightRun - ModuleGap ) / 2 ) - Wall - 2 mm )"
equation "d2503 = ( BaseY ) + ( 10 mm )"
equation "d2506 = PanHeight"
equation "d2508 = ( FootHeight ) - 0.2 mm"
equation "d2510 = ( BaseX ) + ( LeftSideDepth )"
equation "d2511 = ( BaseY + Depth + ModuleGap ) + ( ( LeftReach ) - ( ( -1 mm ) + ( ( LeftReach ) + 2 mm ) ) )"
equation "d2512 = DrainExtension + 2 mm"
equation "d2513 = ( LeftReach ) + 2 mm"
equation "d2514 = PanHeight + 0.4 mm"
equation "d2516 = ( BaseY + Depth + ModuleGap ) + ( ( LeftReach ) - ( Wall ) )"
equation "d2518 = ( ( BaseX ) + ( ( LeftSideDepth ) - Wall - 0.1 mm ) )"
equation "d2519 = -( -( ( FootHeight ) + FloorMin + DrainExtension * tan(DrainSlope) + ( ( LeftSideDepth ) - ( ( LeftSideDepth ) - Wall - 0.1 mm ) ) * tan(DrainSlope) ) )"
equation "d2520 = ( ( BaseX ) + ( ( LeftSideDepth ) + 1 mm ) )"
equation "d2521 = -( -( ( FootHeight ) + FloorMin + DrainExtension * tan(DrainSlope) + ( ( LeftSideDepth ) - ( ( LeftSideDepth ) + 1 mm ) ) * tan(DrainSlope) ) )"
equation "d2522 = -( -( ( FootHeight ) + PanHeight + 1 mm ) )"
equation "d2523 = -( -( -( ( LeftReach ) - 2 * Wall ) ) )"
equation "d2525 = ( FootHeight ) + PanHeight - DeckThick"
equation "d2527 = ( BaseX ) + ( 10 mm - DeckClearance )"
equation "d2528 = ( BaseY + Depth + ModuleGap ) + ( ( LeftReach ) - ( ( ( Wall ) - DeckClearance ) + ( 2 mm + 2 * DeckClearance ) ) )"
equation "d2529 = 5 mm + 2 * DeckClearance"
equation "d2530 = 2 mm + 2 * DeckClearance"
equation "d2531 = DeckThick"
equation "d2533 = FootHeight"
equation "d2535 = ( BaseX ) + ( 10 mm )"
equation "d2536 = ( BaseY + Depth + ModuleGap ) + ( ( LeftReach ) - ( ( Wall ) + ( 2 mm ) ) )"
equation "d2539 = PanHeight"
equation "d2541 = ( FootHeight ) + PanHeight - DeckThick"
equation "d2543 = ( BaseX ) + ( 10 mm - DeckClearance )"
equation "d2544 = ( BaseY + Depth + ModuleGap ) + ( ( LeftReach ) - ( ( ( ( LeftReach ) - Wall - 2 mm ) - DeckClearance ) + ( 2 mm + 2 * DeckClearance ) ) )"
equation "d2545 = 5 mm + 2 * DeckClearance"
equation "d2546 = 2 mm + 2 * DeckClearance"
equation "d2547 = DeckThick"
equation "d2549 = FootHeight"
equation "d2551 = ( BaseX ) + ( 10 mm )"
equation "d2552 = ( BaseY + Depth + ModuleGap ) + ( ( LeftReach ) - ( ( ( LeftReach ) - Wall - 2 mm ) + ( 2 mm ) ) )"
equation "d2555 = PanHeight"
equation "d2557 = ( FootHeight ) - 0.2 mm"
equation "d2559 = ( BaseX + LeftRun + FaucetGap + RightRun - RightSideDepth ) + ( ( RightSideDepth ) - ( ( RightSideDepth ) + ( DrainExtension + 2 mm ) ) )"
equation "d2560 = ( BaseY + Depth + ModuleGap ) + ( -1 mm )"
equation "d2561 = DrainExtension + 2 mm"
equation "d2562 = ( RightReach ) + 2 mm"
equation "d2563 = PanHeight + 0.4 mm"
equation "d2565 = ( BaseY + Depth + ModuleGap ) + ( Wall )"
equation "d2567 = ( ( BaseX + LeftRun + FaucetGap + RightRun - RightSideDepth ) + ( ( RightSideDepth ) - ( ( RightSideDepth ) - Wall - 0.1 mm ) ) )"
equation "d2568 = -( -( ( FootHeight ) + FloorMin + DrainExtension * tan(DrainSlope) + ( ( RightSideDepth ) - ( ( RightSideDepth ) - Wall - 0.1 mm ) ) * tan(DrainSlope) ) )"
equation "d2569 = ( ( BaseX + LeftRun + FaucetGap + RightRun - RightSideDepth ) + ( ( RightSideDepth ) - ( ( RightSideDepth ) + 1 mm ) ) )"
equation "d2570 = -( -( ( FootHeight ) + FloorMin + DrainExtension * tan(DrainSlope) + ( ( RightSideDepth ) - ( ( RightSideDepth ) + 1 mm ) ) * tan(DrainSlope) ) )"
equation "d2571 = -( -( ( FootHeight ) + PanHeight + 1 mm ) )"
equation "d2572 = ( RightReach ) - 2 * Wall"
equation "d2574 = ( FootHeight ) + PanHeight - DeckThick"
equation "d2576 = ( BaseX + LeftRun + FaucetGap + RightRun - RightSideDepth ) + ( ( RightSideDepth ) - ( ( 10 mm - DeckClearance ) + ( 5 mm + 2 * DeckClearance ) ) )"
equation "d2577 = ( BaseY + Depth + ModuleGap ) + ( ( Wall ) - DeckClearance )"
equation "d2578 = 5 mm + 2 * DeckClearance"
equation "d2579 = 2 mm + 2 * DeckClearance"
equation "d2580 = DeckThick"
equation "d2582 = FootHeight"
equation "d2584 = ( BaseX + LeftRun + FaucetGap + RightRun - RightSideDepth ) + ( ( RightSideDepth ) - ( ( 10 mm ) + ( 5 mm ) ) )"
equation "d2585 = ( BaseY + Depth + ModuleGap ) + ( Wall )"
equation "d2588 = PanHeight"
equation "d2590 = ( FootHeight ) + PanHeight - DeckThick"
equation "d2592 = ( BaseX + LeftRun + FaucetGap + RightRun - RightSideDepth ) + ( ( RightSideDepth ) - ( ( 10 mm - DeckClearance ) + ( 5 mm + 2 * DeckClearance ) ) )"
equation "d2593 = ( BaseY + Depth + ModuleGap ) + ( ( ( RightReach ) - Wall - 2 mm ) - DeckClearance )"
equation "d2594 = 5 mm + 2 * DeckClearance"
equation "d2595 = 2 mm + 2 * DeckClearance"
equation "d2596 = DeckThick"
equation "d2598 = FootHeight"
equation "d2600 = ( BaseX + LeftRun + FaucetGap + RightRun - RightSideDepth ) + ( ( RightSideDepth ) - ( ( 10 mm ) + ( 5 mm ) ) )"
equation "d2601 = ( BaseY + Depth + ModuleGap ) + ( ( RightReach ) - Wall - 2 mm )"
equation "d2604 = PanHeight"
equation "d2606 = ( UpperDeckHeight - PanHeight ) - 0.2 mm"
equation "d2608 = ( BaseX ) + ( -1 mm )"
equation "d2609 = ( BaseY ) + ( Depth )"
equation "d2610 = ( TowerWidth ) + 2 mm"
equation "d2611 = DrainExtension + 2 mm"
equation "d2612 = PanHeight + 0.4 mm"
equation "d2614 = ( BaseX ) + ( Wall )"
equation "d2616 = -( -( ( UpperDeckHeight - PanHeight ) + FloorMin + DrainExtension * tan(DrainSlope) + ( ( Depth ) - ( ( Depth ) - Wall - 0.1 mm ) ) * tan(DrainSlope) ) )"
equation "d2617 = ( ( BaseY ) + ( ( Depth ) - Wall - 0.1 mm ) )"
equation "d2618 = -( -( ( UpperDeckHeight - PanHeight ) + FloorMin + DrainExtension * tan(DrainSlope) + ( ( Depth ) - ( ( Depth ) + 1 mm ) ) * tan(DrainSlope) ) )"
equation "d2619 = ( ( BaseY ) + ( ( Depth ) + 1 mm ) )"
equation "d2620 = -( -( ( UpperDeckHeight - PanHeight ) + PanHeight + 1 mm ) )"
equation "d2621 = ( TowerWidth ) - 2 * Wall"
equation "d2623 = ( UpperDeckHeight - PanHeight ) + PanHeight - DeckThick"
equation "d2625 = ( BaseX ) + ( ( Wall ) - DeckClearance )"
equation "d2626 = ( BaseY ) + ( 13 mm - DeckClearance )"
equation "d2627 = 2 mm + 2 * DeckClearance"
equation "d2628 = 5 mm + 2 * DeckClearance"
equation "d2629 = DeckThick"
equation "d2631 = UpperDeckHeight - PanHeight"
equation "d2633 = ( BaseX ) + ( Wall )"
equation "d2634 = ( BaseY ) + ( 13 mm )"
equation "d2637 = PanHeight"
equation "d2639 = ( UpperDeckHeight - PanHeight ) + PanHeight - DeckThick"
equation "d2641 = ( BaseX ) + ( ( ( TowerWidth ) - Wall - 2 mm ) - DeckClearance )"
equation "d2642 = ( BaseY ) + ( 13 mm - DeckClearance )"
equation "d2643 = 2 mm + 2 * DeckClearance"
equation "d2644 = 5 mm + 2 * DeckClearance"
equation "d2645 = DeckThick"
equation "d2647 = UpperDeckHeight - PanHeight"
equation "d2649 = ( BaseX ) + ( ( TowerWidth ) - Wall - 2 mm )"
equation "d2650 = ( BaseY ) + ( 13 mm )"
equation "d2653 = PanHeight"
equation "TouchChamfer = 0.4 mm" comment "R03 selected touch edges; excludes drainage lip and locator bearing faces"
equation "RunnerWidth = 8 mm" comment "R03 integral support rail thickness"
equation "d2657 = FootHeight"
equation "d2659 = ( BaseX + TowerWidth + ModuleGap ) + ( ( 11 mm ) - PegSize / 2 - FitClearance )"
equation "d2660 = ( BaseY ) + ( ( 11 mm ) - PegSize / 2 - FitClearance )"
equation "d2661 = PegSize + 2 * FitClearance"
equation "d2662 = PegSize + 2 * FitClearance"
equation "d2663 = PegHeight + 0.3 mm"
equation "d2665 = FootHeight"
equation "d2667 = ( BaseX + TowerWidth + ModuleGap ) + ( ( 11 mm ) - PegSize / 2 - FitClearance )"
equation "d2668 = ( BaseY ) + ( ( ( Depth ) - FrontFootInset ) - PegSize / 2 - FitClearance )"
equation "d2669 = PegSize + 2 * FitClearance"
equation "d2670 = PegSize + 2 * FitClearance"
equation "d2671 = PegHeight + 0.3 mm"
equation "d2673 = FootHeight"
equation "d2675 = ( BaseX + TowerWidth + ModuleGap ) + ( ( ( LeftRun - TowerWidth - ModuleGap ) - 11 mm ) - PegSize / 2 - FitClearance )"
equation "d2676 = ( BaseY ) + ( ( 11 mm ) - PegSize / 2 - FitClearance )"
equation "d2677 = PegSize + 2 * FitClearance"
equation "d2678 = PegSize + 2 * FitClearance"
equation "d2679 = PegHeight + 0.3 mm"
equation "d2681 = FootHeight"
equation "d2683 = ( BaseX + TowerWidth + ModuleGap ) + ( ( ( LeftRun - TowerWidth - ModuleGap ) - 11 mm ) - PegSize / 2 - FitClearance )"
equation "d2684 = ( BaseY ) + ( ( ( Depth ) - FrontFootInset ) - PegSize / 2 - FitClearance )"
equation "d2685 = PegSize + 2 * FitClearance"
equation "d2686 = PegSize + 2 * FitClearance"
equation "d2687 = PegHeight + 0.3 mm"
equation "d2691 = ( BaseX + TowerWidth + ModuleGap ) + ( 3 mm )"
equation "d2692 = ( BaseY ) + ( 0 mm )"
equation "d2693 = RunnerWidth"
equation "d2694 = ( Depth ) - 9 mm"
equation "d2695 = FootHeight"
equation "d2699 = ( BaseX + TowerWidth + ModuleGap ) + ( ( LeftRun - TowerWidth - ModuleGap ) - 3 mm - RunnerWidth )"
equation "d2700 = ( BaseY ) + ( 0 mm )"
equation "d2701 = RunnerWidth"
equation "d2702 = ( Depth ) - 9 mm"
equation "d2703 = FootHeight"
equation "d2705 = TouchChamfer"
equation "d2706 = FootHeight"
equation "d2708 = ( BaseX + TowerFrame + TowerClearance ) + ( ( 11 mm ) - PegSize / 2 - FitClearance )"
equation "d2709 = ( BaseY ) + ( ( 11 mm ) - PegSize / 2 - FitClearance )"
equation "d2710 = PegSize + 2 * FitClearance"
equation "d2711 = PegSize + 2 * FitClearance"
equation "d2712 = PegHeight + 0.3 mm"
equation "d2714 = FootHeight"
equation "d2716 = ( BaseX + TowerFrame + TowerClearance ) + ( ( 11 mm ) - PegSize / 2 - FitClearance )"
equation "d2717 = ( BaseY ) + ( ( ( Depth ) - FrontFootInset ) - PegSize / 2 - FitClearance )"
equation "d2718 = PegSize + 2 * FitClearance"
equation "d2719 = PegSize + 2 * FitClearance"
equation "d2720 = PegHeight + 0.3 mm"
equation "d2722 = FootHeight"
equation "d2724 = ( BaseX + TowerFrame + TowerClearance ) + ( ( ( TowerWidth - 2 * ( TowerFrame + TowerClearance ) ) - 11 mm ) - PegSize / 2 - FitClearance )"
equation "d2725 = ( BaseY ) + ( ( 11 mm ) - PegSize / 2 - FitClearance )"
equation "d2726 = PegSize + 2 * FitClearance"
equation "d2727 = PegSize + 2 * FitClearance"
equation "d2728 = PegHeight + 0.3 mm"
equation "d2730 = FootHeight"
equation "d2732 = ( BaseX + TowerFrame + TowerClearance ) + ( ( ( TowerWidth - 2 * ( TowerFrame + TowerClearance ) ) - 11 mm ) - PegSize / 2 - FitClearance )"
equation "d2733 = ( BaseY ) + ( ( ( Depth ) - FrontFootInset ) - PegSize / 2 - FitClearance )"
equation "d2734 = PegSize + 2 * FitClearance"
equation "d2735 = PegSize + 2 * FitClearance"
equation "d2736 = PegHeight + 0.3 mm"
equation "d2740 = BaseX"
equation "d2741 = BaseY"
equation "d2742 = TowerFrame"
equation "d2743 = Depth"
equation "d2744 = UpperDeckHeight - PanHeight + 2 mm"
equation "d2748 = BaseX + TowerWidth - TowerFrame"
equation "d2749 = BaseY"
equation "d2750 = TowerFrame"
equation "d2751 = Depth"
equation "d2752 = UpperDeckHeight - PanHeight + 2 mm"
equation "d2754 = FootHeight"
equation "d2756 = BaseX + TowerFrame"
equation "d2757 = BaseY"
equation "d2758 = TowerClearance"
equation "d2759 = Depth"
equation "d2760 = PanHeight"
equation "d2762 = FootHeight"
equation "d2764 = BaseX + TowerWidth - TowerFrame - TowerClearance"
equation "d2765 = BaseY"
equation "d2766 = TowerClearance"
equation "d2767 = Depth"
equation "d2768 = PanHeight"
equation "d2770 = TouchChamfer"
equation "d2771 = FootHeight"
equation "d2773 = ( BaseX + LeftRun + FaucetGap ) + ( ( 11 mm ) - PegSize / 2 - FitClearance )"
equation "d2774 = ( BaseY ) + ( ( 11 mm ) - PegSize / 2 - FitClearance )"
equation "d2775 = PegSize + 2 * FitClearance"
equation "d2776 = PegSize + 2 * FitClearance"
equation "d2777 = PegHeight + 0.3 mm"
equation "d2779 = FootHeight"
equation "d2781 = ( BaseX + LeftRun + FaucetGap ) + ( ( 11 mm ) - PegSize / 2 - FitClearance )"
equation "d2782 = ( BaseY ) + ( ( ( Depth ) - FrontFootInset ) - PegSize / 2 - FitClearance )"
equation "d2783 = PegSize + 2 * FitClearance"
equation "d2784 = PegSize + 2 * FitClearance"
equation "d2785 = PegHeight + 0.3 mm"
equation "d2787 = FootHeight"
equation "d2789 = ( BaseX + LeftRun + FaucetGap ) + ( ( ( ( RightRun - ModuleGap ) / 2 ) - 11 mm ) - PegSize / 2 - FitClearance )"
equation "d2790 = ( BaseY ) + ( ( 11 mm ) - PegSize / 2 - FitClearance )"
equation "d2791 = PegSize + 2 * FitClearance"
equation "d2792 = PegSize + 2 * FitClearance"
equation "d2793 = PegHeight + 0.3 mm"
equation "d2795 = FootHeight"
equation "d2797 = ( BaseX + LeftRun + FaucetGap ) + ( ( ( ( RightRun - ModuleGap ) / 2 ) - 11 mm ) - PegSize / 2 - FitClearance )"
equation "d2798 = ( BaseY ) + ( ( ( Depth ) - FrontFootInset ) - PegSize / 2 - FitClearance )"
equation "d2799 = PegSize + 2 * FitClearance"
equation "d2800 = PegSize + 2 * FitClearance"
equation "d2801 = PegHeight + 0.3 mm"
equation "d2805 = ( BaseX + LeftRun + FaucetGap ) + ( 3 mm )"
equation "d2806 = ( BaseY ) + ( 0 mm )"
equation "d2807 = RunnerWidth"
equation "d2808 = ( Depth ) - 9 mm"
equation "d2809 = FootHeight"
equation "d2813 = ( BaseX + LeftRun + FaucetGap ) + ( ( ( RightRun - ModuleGap ) / 2 ) - 3 mm - RunnerWidth )"
equation "d2814 = ( BaseY ) + ( 0 mm )"
equation "d2815 = RunnerWidth"
equation "d2816 = ( Depth ) - 9 mm"
equation "d2817 = FootHeight"